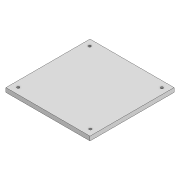
# Autodesk Inventor part: Base
Saved by Autodesk Inventor 2020 (Build 240168000, 168)
## iProperties
Created: 2020-11-07
Part Number: Base
Material: Generic
Document SubType Name: Modeling
Designer: ferrerx
Density: 1 g/cm^3
Appearance: Default
Author: ferrerx
Autodesk Inventor part; units mm, degrees
ref_plane "YZ Plane" through (0, 0, 0) normal (1, 0, 0) x (0, 1, 0)
ref_plane "XZ Plane" through (0, 0, 0) normal (0, 1, 0) x (-1, 0, 0)
ref_plane "XY Plane" through (0, 0, 0) normal (0, 0, 1) x (1, 0, 0)
sketch "Sketch1" plane through (0, 0, 0) normal (0, 1, 0) x (-1, 0, 0)
  line L0 (0, 0) -> (100, 0)
  line L1 (100, 0) -> (100, -100)
  line L2 (100, -100) -> (0, -100)
  line L3 (0, -100) -> (0, 0)
  line L4 (100, -50) -> (0, -50) construction
  line L5 (7.1, -7.5) -> (92.9, -7.5) construction
  line L6 (92.9, -7.5) -> (92.9, -92.5) construction
  line L7 (92.9, -92.5) -> (7.1, -92.5) construction
  line L8 (7.1, -92.5) -> (7.1, -7.5) construction
  line L9 (7.1, -7.5) -> (92.9, -92.5) construction
  line L10 (92.9, -7.5) -> (7.1, -92.5) construction
  circle A0 centre (92.9, -7.5) radius 1.5
  circle A1 centre (92.9, -92.5) radius 1.5
  circle A2 centre (7.1, -92.5) radius 1.5
  circle A3 centre (7.1, -7.5) radius 1.5
  point P0 (50, -50)
  dimension "d0" = 100
  dimension "d1" = 100
  dimension "d2" = 85.8
  dimension "d3" = 85
  dimension "d4" = 3
  dimension "d5" = 3
  dimension "d6" = 3
  dimension "d7" = 3
  constraints: 22 end point, 5 midpoint, 4 centre point, 4 coincident, 4 parallel, 2 horizontal, 2 perpendicular
  measures "d0" distance of L1.end L2.end
  measures "d1" distance of L0.end L1.end
  measures "d2" distance of L6.end L7.end
  measures "d3" distance of L7.end L5.start
  measures "d4" diameter of A1
  measures "d5" diameter of A0
  measures "d6" diameter of A3
  measures "d7" diameter of A2
extrude "Extrusion1" add sketch "Sketch1" along normal blind 5
sketch "Sketch2" plane through (0, 5, 0) normal (0, 1, 0) x (1, 0, 0)
  line L0 (-100, 100) -> (-100, 0) projected
  line L1 (-100, 30) -> (-97, 30)
  line L2 (-97, 30) -> (-97, 70)
  line L3 (-97, 70) -> (-100, 70)
  line L4 (-100, 70) -> (-100, 30)
  line L5 (-97, 50) -> (-100, 50) construction
  line L6 (0, 0) -> (0, 100) projected
  line L7 (0, 50) -> (-100, 50) construction
  line L8 (-100, 0) -> (0, 0) projected
  line L9 (-50, 0) -> (-50, 98) construction
  line L10 (-70, 0) -> (-30, 0)
  line L11 (-30, 0) -> (-30, 3)
  line L12 (-30, 3) -> (-70, 3)
  line L13 (-70, 3) -> (-70, 0)
  line L14 (-50, 3) -> (-50, 0) construction
  line L15 (0, 30) -> (-3, 30)
  line L16 (-3, 30) -> (-3, 70)
  line L17 (-3, 70) -> (0, 70)
  line L18 (0, 70) -> (0, 30)
  line L19 (-3, 50) -> (0, 50) construction
  line L20 (-70, 100) -> (-30, 100)
  line L21 (-30, 100) -> (-30, 97)
  line L22 (-30, 97) -> (-70, 97)
  line L23 (-70, 97) -> (-70, 100)
  line L24 (-50, 97) -> (-50, 100) construction
  dimension "d10" = 40
  dimension "d11" = 3
  dimension "d12" = 40
  dimension "d13" = 3
  constraints: 44 end point, 14 symmetric about line, 7 midpoint, 4 parallel, 3 perpendicular, 2 collinear, 2 horizontal, 2 point on line, 1 vertical
  measures "d10" distance of L1.end L2.end
  measures "d11" distance of L2.end L3.end
  measures "d12" distance between parallel lines of L11 L13
  measures "d13" distance of L10.end L11.end
extrude "Extrusion2" [suppressed]
body "Solid1"
